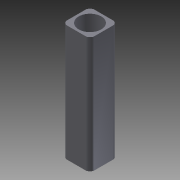
# Autodesk Inventor part: PZT_Guide
Saved by Autodesk Inventor 2011 SP2 (Build 150309200, 309)
## iProperties
Created: 2011-09-20
Part Number: PZT_Guide
Document SubType Name: Modeling
Designer: sungwook
Density: 8.08 g/cm^3
Material: Stainless Steel
Author: sungwook
Autodesk Inventor part; units mm, degrees
ref_plane "YZ Plane" through (0, 0, 0) normal (1, 0, 0) x (0, 1, 0)
ref_plane "XZ Plane" through (0, 0, 0) normal (0, 1, 0) x (-1, 0, 0)
ref_plane "XY Plane" through (0, 0, 0) normal (0, 0, 1) x (1, 0, 0)
sketch "Sketch1" plane through (0, 0, 0) normal (0, 0, 1) x (1, 0, 0)
  line L0 (-0.705, 0.705) -> (0.705, 0.705)
  line L1 (0.705, 0.705) -> (0.705, -0.705)
  line L2 (0.705, -0.705) -> (-0.705, -0.705)
  line L3 (-0.705, -0.705) -> (-0.705, 0.705)
  point P0 (0, 0)
  point P1 (-0.705, 0)
  point P2 (0, 0.705)
  dimension "d0" = 1.41
  constraints: 8 end point, 2 midpoint, 2 parallel, 2 perpendicular, 1 horizontal, 1 horizontal alignment, 1 vertical alignment
  measures "d0" distance of L0.start L0.end
extrude "Extrusion1" add sketch "Sketch1" along normal mid plane 5.97
fillet "Fillet1" [suppressed]
sketch "Sketch2" plane through (0, 0, 2.985) normal (0, 0, 1) x (1, 0, 0)
  circle A0 centre (0, 0) radius 0.58
  dimension "d4" = 1.16
  constraints: 1 centre point, 1 coincident
  measures "d4" diameter of A0
extrude "Extrusion2" cut sketch "Sketch2" against normal blind 1.943
hole "Hole1" at (0, 0, 1.042) direction (0, 0, -1) diameter 1.1 depth 2.1
thread "Thread1" size "M1.1x0.25" class "6H" standard "ISO Metric profile" full length
sketch "Sketch3" plane through (0, 0, -2.985) normal (0, 0, -1) x (-1, 0, 0)
  circle A0 centre (0, 0) radius 0.58
  dimension "d18" = 1.16
  constraints: 1 centre point, 1 coincident
  measures "d18" diameter of A0
extrude "Extrusion3" cut sketch "Sketch3" against normal up to surface (1.927 mm away)
sketch "Sketch4" plane through (0, 0, -2.985) normal (0, 0, -1) x (-1, 0, 0)
  line L0 (-0.705, 0.705) -> (0.705, 0.705) projected
  line L1 (-0.705, -0.705) -> (-0.705, 0.705) projected
  line L2 (0.705, -0.705) -> (-0.705, -0.705) projected
  line L3 (0.705, 0.705) -> (0.705, -0.705) projected
  arc A0 (-0.535, 0.705) -> (-0.705, 0.535) centre (-0.3189, 0.3189) ccw
  circle A1 centre (0.3189, 0.3189) radius 0.4425
  circle A2 centre (-0.3189, -0.3189) radius 0.4425
  circle A3 centre (0.3189, -0.3189) radius 0.4425
  point P0 (0.535, 0.705)
  point P1 (0.705, 0.535)
  point P2 (0.705, -0.535)
  point P3 (0.535, -0.705)
  point P4 (-0.535, -0.705)
  point P5 (-0.705, -0.535)
  dimension "d22" = 0.17
  dimension "d23" = 0.17
  dimension "d25" = 0.885
  dimension "d26" = 0.885
  dimension "d27" = 0.885
  dimension "d28" = 0.17
  dimension "d29" = 0.17
  dimension "d30" = 0.17
  dimension "d31" = 0.17
  dimension "d32" = 0.17
  dimension "d33" = 0.17
  constraints: 8 point on circle, 8 point on line, 4 centre point
  measures "d22" distance from line of A0.start L1
  measures "d23" distance from line of A0.end L0
  measures "d25" diameter of A1
  measures "d26" diameter of A2
  measures "d27" diameter of A3
  measures "d28" distance from line of A1.start L3
  measures "d29" distance from line of L0 A1.end
  measures "d30" distance from line of L3 A3.end
  measures "d31" distance from line of L2 A3.start
  measures "d32" distance from line of L2 A2.end
  measures "d33" distance from line of L1 A2.start
extrude "Extrusion4" cut sketch "Sketch4" against normal through all contours L0 A0 L1 | L0 L3 A1 | A2 L2 L1 | L3 L2 A3
fillet "Fillet2" radius 0.15 8 edges at (0.705, 0.535, 0) (0.535, 0.705, 0) (-0.535, 0.705, 0) (-0.705, 0.535, 0) (-0.705, -0.535, 0) (-0.535, -0.705, 0) (0.535, -0.705, 0) (0.705, -0.535, 0)
body "Solid1"
